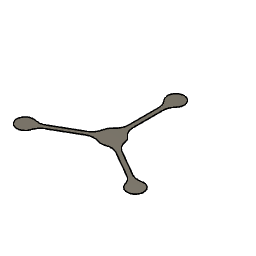
Rostock Leveling Jig v1 (Autodesk Fusion 360 design; units mm, degrees)
Autodesk Fusion 360 part; units mm, degrees
sketch "Sketch1" plane through (0, 0, 0) normal (0, 1, 0) x (1, 0, 0)
  line L0 (0, 130) -> (-112.5833, -65) construction
  line L1 (-112.5833, -65) -> (112.5833, -65) construction
  line L2 (112.5833, -65) -> (0, 130) construction
  line L3 (0, 0) -> (0, 130) construction
  line L4 (0, 0) -> (-112.5833, -65) construction
  line L5 (0, 0) -> (112.5833, -65) construction
  circle A0 centre (0, 115) radius 15
  circle A1 centre (-99.5929, -57.5) radius 15
  circle A2 centre (99.5929, -57.5) radius 15
  circle A3 centre (0, 0) radius 20
  line L6 (-4, 19.5959) -> (4, 19.5959) construction
  line L7 (4, 19.5959) -> (4, 100.5432)
  line L8 (4, 100.5432) -> (-4, 100.5432) construction
  line L9 (-4, 100.5432) -> (-4, 19.5959)
  line L10 (-85.0729, -53.7357) -> (-14.9706, -13.2621)
  line L11 (-18.9706, -6.3339) -> (-89.0729, -46.8075)
  line L12 (89.0729, -46.8075) -> (18.9706, -6.3339)
  line L13 (14.9706, -13.2621) -> (85.0729, -53.7357)
  point P0 (0, 100.5432)
  point P1 (0, 19.5959)
  dimension "d1" = 130
  dimension "d2" = 30
  dimension "d4" = 360
  dimension "d5" = 40
  dimension "d6" = 8
  dimension "d8" = 360
  constraint coincident L3.start L4.start
  constraint horizontal L1
  constraint coincident L2 L0.start
  constraint coincident L0 L2.end
  constraint coincident L3 A0.centre
  constraint coincident L0.start A0
  constraint horizontal L6
  constraint vertical L7
  constraint horizontal L8
  constraint vertical L9
  constraint coincident A3 L6.start
  constraint midpoint L8 P0
  constraint midpoint L6 P1
  constraint coincident L3 P1
  constraint coincident A0 L7.end
  measures "d1" distance of L0.start L3.start
  measures "d2" diameter of A0
  measures "d5" diameter of A3
  measures "d6" distance of L7.end L8.end
extrude "Extrude1" add sketch "Sketch1" along normal blind 0.4
fillet "Fillet1" radius 24 12 edges at (-4, 0.2, -100.5432) (4, 0.2, -100.5432) (-4, 0.2, -19.5959) (4, 0.2, -19.5959) (-18.9706, 0.2, 6.3339) (-14.9706, 0.2, 13.2621) (14.9706, 0.2, 13.2621) (18.9706, 0.2, 6.3339) (85.0729, 0.2, 53.7357) (89.0729, 0.2, 46.8075) (-89.0729, 0.2, 46.8075) (-85.0729, 0.2, 53.7357)
